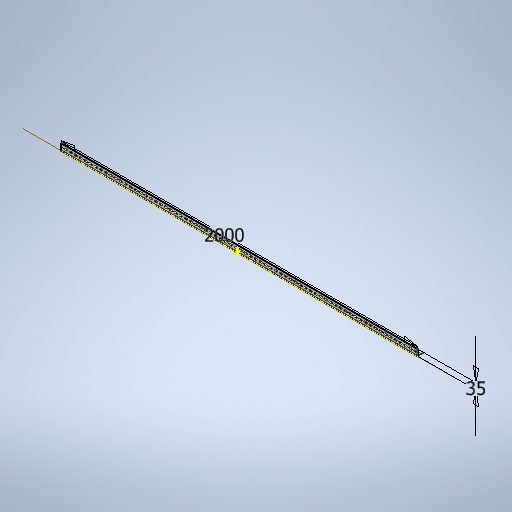
# Autodesk Inventor part: KTP35H35_2_620520
Saved by Autodesk Inventor 2025.2 (Build 292293000, 293)
## iProperties
Created: 2026-04-20
Part Number: KTP35H35_2_620520
Material: Generic
Document SubType Name: Sheet Metal
Designer: Oski
Density: 1 g/cm^3
Sheet Metal Rule: Default_mm
Appearance: Default
Author: Oski
Autodesk Inventor part; units mm, degrees
ref_plane "YZ Plane" through (0, 0, 0) normal (1, 0, 0) x (0, 1, 0)
ref_plane "XZ Plane" through (0, 0, 0) normal (0, 1, 0) x (-1, 0, 0)
ref_plane "XY Plane" through (0, 0, 0) normal (0, 0, 1) x (1, 0, 0)
sketch "Sketch1" plane through (0, 0, 0) normal (0, 0, 1) x (1, 0, 0)
  line L0 (-1000, 17.5) -> (1000, 17.5)
  line L1 (1000, 17.5) -> (1000, -17.5)
  line L2 (1000, -17.5) -> (-1000, -17.5)
  line L3 (-1000, -17.5) -> (-1000, 17.5)
  line L4 (0, 0) -> (0, 17.5) construction
  line L5 (0, 0) -> (0, -17.5) construction
  line L6 (0, 0) -> (-1000, 0) construction
  line L7 (0, 0) -> (1000, 0) construction
  dimension "d1" = 2000
  dimension "d2" = 35
  measures "d1" distance of L0.start L0.end
  measures "d2" distance of L0.end L1.end
extrude "Plate1" add sketch "Sketch1" along normal blind 1.5
sketch "Sketch2" plane through (-1000, -16, 1.5) normal (0, -1, 0) x (1, 0, 0)
  line L0 (2000, 0) -> (0, 0)
  line L1 (0, 0) -> (0, -35)
  line L2 (0, -35) -> (2000, -35)
  line L3 (2000, -35) -> (2000, 0)
  constraints: 6 end point, 1 horizontal, 1 perpendicular, 1 vertical
edge flange "Flange1" height 35 angle 90 thickness 1.5 bend radius 1.5 thickness toward (0, -1, 0) relief straight relief width 1.5 relief depth 0.75 edges at (0, -17.5, 0) wall of the first edge with corners at (1000, -16, 1.5) (-1000, -16, 1.5) (-1000, -16, -33.5) (1000, -16, -33.5)
bend "Bend1"
corner "Corner1"
sketch "Sketch3" plane through (-1000, -16, -33.5) normal (0, 1, 0) x (1, 0, 0)
  line L0 (23.5, -16.5) -> (32.5, -16.5) construction
  line L1 (23.5, -21) -> (32.5, -21)
  line L2 (32.5, -12) -> (23.5, -12)
  arc A0 (23.5, -12) -> (23.5, -21) centre (23.5, -16.5) ccw
  arc A1 (32.5, -21) -> (32.5, -12) centre (32.5, -16.5) ccw
  line L3 (0, -32) -> (0, 0) projected
  line L4 (2000, 0) -> (0, 0) projected
  line L5 (2000, -33.5) -> (2000, -32) projected
  line L6 (2000, 0) -> (2000, -32) construction
  point P0 (1000, -33.5)
  point P1 (28, -16.5)
  point P2 (19, -16.5)
  point P3 (37, -16.5)
  point P4 (28, -21)
  point P5 (28, -12)
  dimension "d15" = 18
  dimension "d16" = 9
  dimension "d17" = 28
  dimension "d18" = 12
  constraints: 10 end point, 6 point on circle, 4 tangent, 3 midpoint, 2 centre point, 1 horizontal, 1 parallel, 1 vertical
  measures "d15" distance of point (19, -16.5) point (37, -16.5)
  measures "d16" distance of point (28, -21) point (28, -12)
  measures "d17" distance from line of L3 point (28, -16.5)
  measures "d18" distance from line of L4 point (28, -12)
extrude "Extrusion1" cut sketch "Sketch3" against normal blind 10
pattern_linear "Rectangular Pattern1" count 71 spacing 28 along (1, 0, 0) of "Extrusion1"
sketch "Sketch5" plane through (0, 0, 1.5) normal (0, 0, 1) x (1, 0, 0)
  line L0 (1000, -17.5) -> (-1000, -17.5) projected
  line L1 (-1000, -17.5) -> (-968.7357, -17.5)
  point P0 (0, 0)
  constraints: 2 end point, 1 point on line
sketch "Sketch6" plane through (-1000, -17.5, -33.5) normal (0, -1, 0) x (1, 0, 0)
  line L0 (2000, 33.5) -> (2000, 35) projected
  line L1 (2000, 35) -> (0, 35)
  point P0 (1000, 33.5)
  constraints: 2 end point, 1 horizontal
pattern_circular "Circular Pattern2" count 2 over 90 about axis through (1000, -17.5, 1.5) along (1, 0, 0) of "Extrusion1", "Rectangular Pattern1"
equation "\"d0\" = Thickness"
equation "\"d3\" = BendReliefWidth"
equation "\"d4\" = BendReliefDepth"
equation "\"d5\" = MinimumRemnant"
equation "\"d6\" = TransitionRadius"
equation "\"d9\" = BendRadius"
equation "\"d10\" = CornerReliefSize"
equation "\"d11\" = GapSize"
equation "\"d12\" = JacobiRadiusSize"
equation "\"BendRadius\" = Thickness"
equation "\"BendReliefWidth\" = Thickness"
equation "\"BendReliefDepth\" = 0.5 * Thickness"
equation "\"CornerReliefSize\" = 4 * Thickness"
equation "\"MinimumRemnant\" = 2 * Thickness"
equation "\"TransitionRadius\" = BendRadius"
equation "\"JacobiRadiusSize\" = BendRadius"
equation "\"GapSize\" = Thickness"
equation "\"Thickness\" = 1.5"
body "Solid1"
